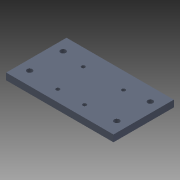
# Autodesk Inventor part: 1_0204_010
Saved by Autodesk Inventor 2012 SP1 (Build 160190100, 190)
## iProperties
Created: 2013-03-27
Part Number: 1_0204_010
Material: Default
Document SubType Name: Modeling
Designer: vogel
Density: 1 g/cm^3
Author: vogel
Autodesk Inventor part; units mm, degrees
ref_plane "YZ Plane" through (0, 0, 0) normal (1, 0, 0) x (0, 1, 0)
ref_plane "XZ Plane" through (0, 0, 0) normal (0, 1, 0) x (-1, 0, 0)
ref_plane "XY Plane" through (0, 0, 0) normal (0, 0, 1) x (1, 0, 0)
sketch "Skizze1" plane through (0, 0, 0) normal (0, 0, 1) x (1, 0, 0)
  line L0 (-80, 25) -> (80, 25)
  line L1 (80, 25) -> (80, -65)
  line L2 (80, -65) -> (-80, -65)
  line L3 (-80, -65) -> (-80, 25)
  line L4 (-112, 0) -> (112, 0) projected
  line L5 (0, -83) -> (0, 43) projected
  circle A0 centre (-30, 0) radius 2.7
  circle A1 centre (30, 0) radius 2.7
  point P0 (0, 0)
  dimension "d0" = 25
  dimension "d1" = 160
  dimension "d2" = 60
  dimension "d3" = 5.4
  dimension "d4" = 90
  constraints: 8 end point, 2 centre point, 2 coincident, 2 parallel, 2 point on line, 1 equal radius, 1 horizontal, 1 perpendicular, 1 symmetric about line, 1 other
  measures "d0" distance between parallel lines of L0 L4
  measures "d1" distance of L0.start L0.end
  measures "d2" distance of point (30, 0) point (-30, 0)
  measures "d3" diameter of A0
  measures "d4" distance of L2.end L0.start
extrude "Extrusion1" add sketch "Skizze1" along normal blind 10 contours L0 L5 L4 A0 L3 | L0 L1 L4 A1 L5 | L4 A0 L5 L2 L3 | L4 A1 L1 L2 L5
sketch "Skizze2" plane through (0, 0, 0) normal (0, 0, -1) x (-1, 0, 0)
  circle A0 centre (-30, 0) radius 2.7 projected
  circle A1 centre (30, 0) radius 2.7 projected
  circle A2 centre (-30, 0) radius 7
  circle A3 centre (30, 0) radius 7
  point P0 (0, 0)
  dimension "d7" = 14
  constraints: 2 centre point, 2 coincident, 1 equal radius
  measures "d7" diameter of A2
extrude "Extrusion2" cut sketch "Skizze2" against normal blind 6
sketch "Skizze3" plane through (0, 0, 0) normal (0, 0, -1) x (-1, 0, 0)
  circle A0 centre (12.5, -59) radius 2.067 projected
  circle A1 centre (-12.5, -59) radius 2.067 projected
  circle A2 centre (-12.5, -37) radius 2.067 projected
  circle A3 centre (12.5, -37) radius 2.067 projected
  line L0 (30, -31) -> (30, -65) projected
  line L1 (30, -65) -> (-30, -65) projected
  line L2 (-30, -65) -> (-30, -31) projected
  line L3 (-30, -31) -> (30, -31) projected
  line L4 (-30, -48) -> (30, -48)
  line L5 (0, -31) -> (0, -65)
  circle A4 centre (-20, -48) radius 2.067 projected
  circle A5 centre (20, -48) radius 2.067 projected
  point P0 (0, 0)
  point P1 (-20, -48)
  point P2 (20, -48)
  dimension "d10" = 40
  constraints: 4 end point, 4 midpoint, 2 point on line, 1 symmetric about line
  measures "d10" distance of point (20, -48) point (-20, -48)
hole "Bohrung1" at (20, -48, 0) at (-20, -48, 0) direction (0, 0, 1) diameter 5.5 end through all counterbore diameter 10 counterbore depth 5.4
sketch "Skizze4" plane through (-80, 25, 0) normal (0, 1, 0) x (1, 0, 0)
  line L0 (0, -10) -> (160, -10) projected
  line L1 (160, 0) -> (160, -10) projected
  line L2 (0, 0) -> (0, -10) projected
  line L3 (160, -5) -> (0, -5)
  line L4 (80, 0) -> (80, -10)
  point P0 (155, -5)
  point P1 (145, -5)
  point P2 (5, -5)
  point P3 (15, -5)
  dimension "d18" = 5
  dimension "d19" = 10
  constraints: 4 end point, 4 point on line, 3 midpoint, 2 symmetric about line
  measures "d18" distance from line of L2 point (5, -5)
  measures "d19" distance of point (5, -5) point (15, -5)
hole "Bohrung2" at (75, 25, 5) at (65, 25, 5) at (-75, 25, 5) at (-65, 25, 5) direction (0, -1, 0) diameter 2.459 depth 10 tip angle 118 thread size "M3x0.5" class "6H" standard "ISO Metric profile"
sketch "Skizze5" plane through (0, 0, 10) normal (0, 0, 1) x (1, 0, 0)
  line L0 (80, 25) -> (80, -65) projected
  line L1 (-80, 25) -> (80, 25) projected
  line L2 (-80, -65) -> (-80, 25) projected
  line L3 (80, -65) -> (-80, -65) projected
  line L4 (0, -65) -> (0, 25)
  line L5 (-80, -20) -> (80, -20)
  line L6 (-65, 5) -> (65, 5)
  line L7 (65, 5) -> (65, -45)
  line L8 (65, -45) -> (-65, -45)
  line L9 (-65, -45) -> (-65, 5)
  point P0 (0, 0)
  dimension "d27" = 130
  dimension "d28" = 50
  constraints: 12 end point, 4 coincident, 4 midpoint, 2 parallel, 1 horizontal, 1 perpendicular, 2 other
  measures "d27" distance of L7.end L8.end
  measures "d28" distance of L8.end L6.start
hole "Bohrung3" at (-65, 5, 10) at (65, 5, 10) at (65, -45, 10) at (-65, -45, 10) direction (0, 0, -1) diameter 4.5 end through all counterbore diameter 8 counterbore depth 6
